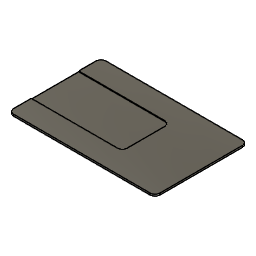
card-adapter (Autodesk Fusion 360 design; units mm, degrees)
Autodesk Fusion 360 part; units mm, degrees
note: some values were not read from the file. Set by a fixed rule: which sketch regions a step uses.
sketch "Sketch1" plane through (0, 0, 0) normal (0, 0, 1) x (1, 0, 0)
  line L0 (0.88, -1.5) -> (80.72, -1.5)
  line L1 (83.6, 1.38) -> (83.6, 49.6)
  line L2 (80.72, 52.48) -> (0.88, 52.48)
  line L3 (-2, 49.6) -> (-2, 1.38)
  arc A0 (-2, 1.38) -> (0.88, -1.5) centre (0.88, 1.38) ccw
  arc A1 (0.88, 52.48) -> (-2, 49.6) centre (0.88, 49.6) ccw
  arc A2 (80.72, -1.5) -> (83.6, 1.38) centre (80.72, 1.38) ccw
  arc A3 (83.6, 49.6) -> (80.72, 52.48) centre (80.72, 49.6) ccw
  point P0 (-2, -1.5)
  point P1 (83.6, -1.5)
  point P2 (-2, 52.48)
  dimension "d1" = 53.98
  dimension "d2" = 85.6
  dimension "d5" = 2.88
  constraint horizontal L0
  constraint vertical L1
  constraint horizontal L2
  constraint vertical L3
  constraint coincident P0 L0
  constraint coincident P0 L3
  constraint tangent L0 A0
  constraint tangent L3 A0
  constraint coincident P2 L2
  constraint coincident P2 L3
  constraint tangent L2 A1
  constraint tangent L3 A1
  constraint equal A0 A1
  constraint coincident P1 L0
  constraint coincident P1 L1
  constraint tangent L0 A2
  constraint tangent L1 A2
  constraint equal A0 A2
  constraint tangent L1 A3
  constraint tangent L2 A3
  constraint equal A0 A3
  measures "d1" distance of P0 P2
  measures "d2" distance of P0 P1
  measures "d5" radius of A0
extrude "Extrude1" add sketch "Sketch1" along normal blind 1
sketch "Sketch2" plane through (0, 0, 1) normal (0, 0, 1) x (-1, 0, 0)
  arc A0 (-83.6, -49.6) -> (-80.72, -52.48) centre (-80.72, -49.6) ccw
  line L0 (-80.72, -52.48) -> (-0.88, -52.48)
  arc A1 (-0.88, -52.48) -> (2, -49.6) centre (-0.88, -49.6) ccw
  line L1 (2, -49.6) -> (2, -1.38)
  arc A2 (2, -1.38) -> (-0.88, 1.5) centre (-0.88, -1.38) ccw
  line L2 (-0.88, 1.5) -> (-80.72, 1.5)
  arc A3 (-80.72, 1.5) -> (-83.6, -1.38) centre (-80.72, -1.38) ccw
  line L3 (-83.6, -1.38) -> (-83.6, -49.6)
  line L4 (2, -11.7075) -> (-48.38, -11.7075)
  line L5 (-51.26, -14.5875) -> (-51.26, -36.5775)
  line L6 (-48.38, -39.4575) -> (2, -39.4575)
  line L7 (2, -39.4575) -> (2, -11.7075)
  arc A4 (-51.26, -36.5775) -> (-48.38, -39.4575) centre (-48.38, -36.5775) ccw
  arc A5 (-48.38, -11.7075) -> (-51.26, -14.5875) centre (-48.38, -14.5875) ccw
  point P0 (-51.26, -11.7075)
  point P1 (-51.26, -39.4575)
  dimension "d6" = 27.75
  dimension "d7" = 13.0225
  dimension "d8" = 53.26
  dimension "d11" = 2.88
  dimension "d12" = 2.88
  constraint horizontal L4
  constraint vertical L5
  constraint horizontal L6
  constraint vertical L7
  constraint coincident L1 L4.start
  constraint coincident P1 L5
  constraint coincident P1 L6
  constraint tangent L5 A4
  constraint tangent L6 A4
  constraint coincident P0 L4
  constraint coincident P0 L5
  constraint tangent L4 A5
  constraint tangent L5 A5
  measures "d6" distance of P0 P1
  measures "d7" distance of L0 L6
  measures "d8" distance of P1 L6.end
  measures "d11" radius of A4
  measures "d12" radius of A5
extrude "Extrude2" cut sketch "Sketch2" against normal blind 0.4 contours L1 L4 L5 L6 L7 A4 A5
